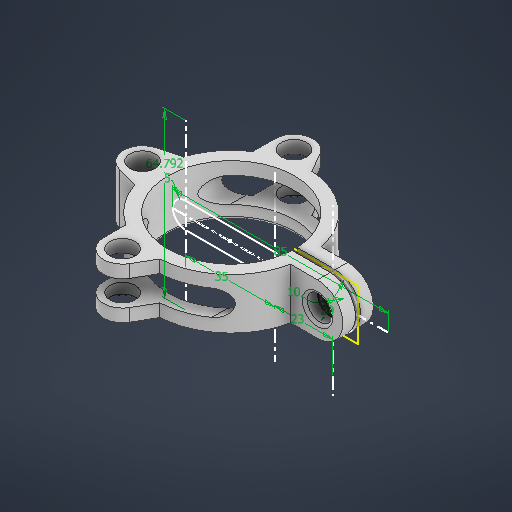
# Autodesk Inventor part: Day02_Task04
Saved by Autodesk Inventor 2026.3 (Build 303398000, 398)
## iProperties
Created: 2026-08-05
Part Number: Day02_Task04
Material: 일반
Document SubType Name: Modeling
Designer: hojin
Density: 1 g/cm^3
Appearance: 기본값
Author: hojin
Autodesk Inventor part; units mm, degrees
ref_plane "YZ Plane" through (0, 0, 0) normal (1, 0, 0) x (0, 1, 0)
ref_plane "XZ Plane" through (0, 0, 0) normal (0, 1, 0) x (-1, 0, 0)
ref_plane "XY Plane" through (0, 0, 0) normal (0, 0, 1) x (1, 0, 0)
sketch "스케치1" plane through (0, 0, 0) normal (0, 1, 0) x (-1, 0, 0)
  arc A0 (-24.98, -1) -> (-24.98, 1) centre (0, 0) ccw
  arc A1 (0, -59.2205) -> (15.3274, -57.2026) centre (0, 0) ccw
  line L0 (0, 0) -> (0, -59.2205) construction
  line L1 (0, 0) -> (15.3274, -57.2026) construction
  arc A2 (2.5635, -37.5574) -> (16.5587, -33.8074) centre (9.0587, -33.8074) ccw
  circle A3 centre (9.0587, -33.8074) radius 5
  line L2 (0, 0) -> (10, 2.6795)
  line L3 (2.5635, -37.5574) -> (-1.8321, -29.944)
  line L4 (16.5587, -33.8074) -> (16.5587, -25.0162)
  arc A4 (36.9411, -7.2444) -> (36.9411, 7.2444) centre (35, 0) ccw
  circle A5 centre (35, 0) radius 5
  line L5 (36.9411, 7.2444) -> (28.4495, 9.5198)
  line L6 (36.9411, -7.2444) -> (28.4495, -9.5198)
  arc A6 (16.5587, 33.8074) -> (2.5635, 37.5574) centre (9.0587, 33.8074) ccw
  circle A7 centre (9.0587, 33.8074) radius 5
  line L7 (2.5635, 37.5574) -> (-1.8321, 29.944)
  line L8 (16.5587, 33.8074) -> (16.5587, 25.0162)
  arc A8 (16.5587, -25.0162) -> (28.4495, -9.5198) centre (0, 0) ccw
  arc A9 (28.4495, 9.5198) -> (16.5587, 25.0162) centre (0, 0) ccw
  line L9 (-50, -6) -> (-29.3939, -6)
  line L10 (-50, 6) -> (-29.3939, 6)
  line L11 (-24.98, 1) -> (-50, 1)
  line L12 (-24.98, -1) -> (-50, -1)
  arc A10 (-1.8321, 29.944) -> (-29.3939, 6) centre (0, 0) ccw
  arc A11 (-29.3939, -6) -> (-1.8321, -29.944) centre (0, 0) ccw
  line L13 (-50, 6) -> (-50, 1)
  line L14 (-50, -1) -> (-50, -6)
  dimension "d0" = 50
  dimension "d2" = 15
  dimension "d4" = 15
  dimension "d5" = 10
  dimension "d6" = 10
  dimension "d7" = 35
  dimension "d10" = 2.6795
  dimension "d18" = 30
  dimension "d24" = 59.2205
  dimension "d29" = 150
  dimension "d31" = 30
  dimension "d32" = 12
  dimension "d34" = 2
  dimension "d35" = 1
  dimension "d36" = 50
  constraints: 30 end point, 18 point on circle, 12 centre point, 6 coincident, 4 perpendicular, 3 concentric, 3 equal length, 2 horizontal, 2 tangent, 2 vertical, 1 point on line, 1 vertical alignment, 23 other
  measures "d0" diameter of A0
  measures "d2" angle of L0 L1
  measures "d4" diameter of A2
  measures "d5" diameter of A3
  measures "d6" horizontal distance of L0.start L2.end
  measures "d7" distance from line of L2 A3.centre
  measures "d10" vertical distance of L0.start L2.end
  measures "d18" angle of L3 L4
  measures "d24" distance of L0.end point (0, 0)
  measures "d31" radius of A8
  measures "d32" distance of L10.start L9.start
  measures "d34" distance between parallel lines of L11 L12
  measures "d35" distance from line of L12 point (0, 0)
  measures "d36" distance between parallel lines of L0 L14
extrude "돌출1" add sketch "스케치1" along normal blind 20
sketch "스케치2" plane through (0, 0, 0) normal (0, 0, 1) x (1, 0, 0)
  circle A0 centre (40, 10) radius 10
  line L0 (50, 0) -> (50, 20) projected
  line L1 (50, 0) -> (24.98, 0) projected
  circle A1 centre (40, 10) radius 5
  line L2 (17, 42.3962) -> (17, -22.3962)
  line L3 (-18, 42.3962) -> (-18, -22.3962)
  line L4 (40, 42.3962) -> (40, -22.3962)
  line L5 (62, 10) -> (-23, 10)
  line L6 (17, 10) -> (-18, 10) construction
  line L7 (17, 5) -> (-18, 5)
  line L8 (-18, 15) -> (17, 15)
  arc A2 (17, 5) -> (17, 15) centre (17, 10) ccw
  arc A3 (-18, 15) -> (-18, 5) centre (-18, 10) ccw
  line L9 (24.98, 20) -> (50, 20) projected
  line L10 (40, 20) -> (50, 20)
  line L11 (50, 20) -> (50, 0)
  point P0 (0, 0)
  point P1 (-0.5, 10)
  dimension "d39" = 20
  dimension "d40" = 10
  dimension "d41" = 23
  dimension "d42" = 35
  dimension "d43" = 85
  dimension "d44" = 5
  dimension "d45" = 64.7924
  constraints: 20 end point, 5 point on circle, 4 horizontal alignment, 4 midpoint, 4 point on line, 4 tangent, 4 vertical, 3 centre point, 2 horizontal, 1 coincident, 1 parallel, 1 perpendicular, 1 vertical alignment, 3 other
  measures "d40" diameter of A1
  measures "d41" distance between parallel lines of L2 L4
  measures "d42" distance between parallel lines of L3 L2
  measures "d43" distance of L5.start L5.end
  measures "d44" radius of A3
  measures "d45" distance of L3.start L3.end
extrude "돌출2" cut sketch "스케치2" along normal blind 100 and the other way blind 30 contours A2 L5 L2 | L2 L5 L3 L8 | L5 A2 L2 | L2 L7 L3 L5 | L3 L5 A3 | L3 A3 L5
extrude "돌출3" cut sketch "스케치2" along normal mid plane 100 contours A2 L5 L2 | L2 L5 L3 L8 | L5 A2 L2 | L2 L7 L3 L5 | L3 L5 A3 | L3 A3 L5
extrude "돌출4" cut sketch "스케치2" along normal mid plane 100 contours L5 L4 A1 | A1 L4 L5 | L4 L5 A1 | A1 L5 L4
fillet "모깎기1" radius 10 4 edges at (50, 0, 3.5) (50, 0, -3.5) (50, 20, -3.5) (50, 20, 3.5)
fillet "모깎기2" radius 1 6 edges at (-4.0587, 0, 33.8074) (-25, 0, 0) (-30, 0, 0) (-4.0587, 0, -33.8074) (35, 10, 6) (35, 10, -6)
